Autodesk Inventor part; units mm, degrees
(part 4 of 5)
sketch "Эскиз44" plane through (1.5, 0, 0) normal (1, 0, 0) x (0, 0, -1)
  arc A0 (42, 27.152) -> (40, 25.152) centre (42, 25.152) ccw projected
  line L0 (40, 25.152) -> (40, 3) projected
  arc A1 (37, 0) -> (40, 3) centre (37, 3) ccw projected
  line L1 (37, 0) -> (-7, 0) projected
  arc A2 (-10, 3) -> (-7, 0) centre (-7, 3) ccw projected
  line L2 (-10, 3) -> (-10, 160) projected
  arc A3 (-7, 163) -> (-10, 160) centre (-7, 160) ccw projected
  line L3 (-7, 163) -> (37, 163) projected
  arc A4 (40, 160) -> (37, 163) centre (37, 160) ccw projected
  line L4 (40, 160) -> (40, 109.152) projected
  arc A5 (40, 109.152) -> (42, 107.152) centre (42, 109.152) ccw projected
  line L5 (42, 107.152) -> (54, 107.152) projected
  arc A6 (56, 105.152) -> (54, 107.152) centre (54, 105.152) ccw projected
  line L6 (56, 105.152) -> (56, 29.152) projected
  arc A7 (54, 27.152) -> (56, 29.152) centre (54, 29.152) ccw projected
  line L7 (54, 27.152) -> (42, 27.152) projected
  circle A8 centre (383.6, 368.9) radius 1.625 projected
  circle A9 centre (-13.6, 369) radius 1.625 projected
  circle A10 centre (383.6, 1.1) radius 1.625 projected
  circle A11 centre (-13.6, 1.1) radius 1.625 projected
  circle A12 centre (379.0468, 185.0848) radius 1.625 projected
  circle A13 centre (-9.0468, 185.0848) radius 1.625 projected
  circle A14 centre (379, 228) radius 1.625 projected
  circle A15 centre (-9, 228) radius 1.625 projected
  arc A16 (315.125, 369.3693) -> (315.125, 366.6307) centre (314.25, 368) ccw projected
  arc A17 (315.125, 366.6307) -> (315.125, 369.3693) centre (316, 368) ccw projected
  arc A18 (298.125, 229.3693) -> (298.125, 226.6307) centre (297.25, 228) ccw projected
  arc A19 (298.125, 226.6307) -> (298.125, 229.3693) centre (299, 228) ccw projected
  circle A20 centre (54, 228) radius 1.625 projected
  circle A21 centre (71, 142) radius 1.625 projected
  circle A22 centre (71, 2.0002) radius 1.625 projected
  circle A23 centre (54, 2.0002) radius 1.625 projected
  circle A24 centre (71, 368) radius 1.625 projected
  circle A25 centre (71, 228) radius 1.625 projected
  arc A26 (315.125, 143.3693) -> (315.125, 140.6307) centre (314.25, 142) ccw projected
  arc A27 (315.125, 140.6307) -> (315.125, 143.3693) centre (316, 142) ccw projected
  arc A28 (315.125, 229.3693) -> (315.125, 226.6307) centre (314.25, 228) ccw projected
  arc A29 (315.125, 226.6307) -> (315.125, 229.3693) centre (316, 228) ccw projected
  circle A30 centre (183.175, 129.0059) radius 1.85 projected
  arc A31 (298.125, 369.3693) -> (298.125, 366.6307) centre (297.25, 368) ccw projected
  arc A32 (298.125, 366.6307) -> (298.125, 369.3693) centre (299, 368) ccw projected
  arc A33 (315.125, 3.3695) -> (315.125, 0.6309) centre (314.25, 2.0002) ccw projected
  arc A34 (315.125, 0.6309) -> (315.125, 3.3695) centre (316, 2.0002) ccw projected
  circle A35 centre (54, 142) radius 1.625 projected
  circle A36 centre (54, 368) radius 1.625 projected
  arc A37 (298.125, 3.3695) -> (298.125, 0.6309) centre (297.25, 2.0002) ccw projected
  arc A38 (298.125, 0.6309) -> (298.125, 3.3695) centre (299, 2.0002) ccw projected
  arc A39 (298.125, 143.3693) -> (298.125, 140.6307) centre (297.25, 142) ccw projected
  arc A40 (298.125, 140.6307) -> (298.125, 143.3693) centre (299, 142) ccw projected
  arc A41 (185, 193.309) -> (185, 192.7028) centre (183.175, 193.0059) ccw projected
  line L8 (185, 193.309) -> (185, 192.7028) projected
  line L9 (14.5, 247.5001) -> (35, 247.5001) projected
  arc A42 (38, 244.5001) -> (35, 247.5001) centre (35, 244.5001) ccw projected
  line L10 (38, 244.5001) -> (38, 185.5001) projected
  arc A43 (35, 182.5001) -> (38, 185.5001) centre (35, 185.5001) ccw projected
  line L11 (35, 182.5001) -> (14.5, 182.5001) projected
  arc A44 (11.5, 185.5001) -> (14.5, 182.5001) centre (14.5, 185.5001) ccw projected
  line L12 (11.5, 185.5001) -> (11.5, 244.5001) projected
  arc A45 (14.5, 247.5001) -> (11.5, 244.5001) centre (14.5, 244.5001) ccw projected
  line L13 (358.5, 244.5001) -> (358.5, 185.5001) projected
  arc A46 (355.5, 182.5001) -> (358.5, 185.5001) centre (355.5, 185.5001) ccw projected
  line L14 (355.5, 182.5001) -> (335, 182.5001) projected
  arc A47 (332, 185.5001) -> (335, 182.5001) centre (335, 185.5001) ccw projected
  line L15 (332, 185.5001) -> (332, 244.5001) projected
  arc A48 (335, 247.5001) -> (332, 244.5001) centre (335, 244.5001) ccw projected
  line L16 (335, 247.5001) -> (355.5, 247.5001) projected
  arc A49 (358.5, 244.5001) -> (355.5, 247.5001) centre (355.5, 244.5001) ccw projected
  line L17 (98.825, 226.3849) -> (98.825, 137.3849) projected
  arc A50 (95.825, 134.3849) -> (98.825, 137.3849) centre (95.825, 137.3849) ccw projected
  line L18 (95.825, 134.3849) -> (87.825, 134.3849) projected
  arc A51 (84.825, 137.3849) -> (87.825, 134.3849) centre (87.825, 137.3849) ccw projected
  line L19 (84.825, 137.3849) -> (84.825, 226.3849) projected
  arc A52 (87.825, 229.3849) -> (84.825, 226.3849) centre (87.825, 226.3849) ccw projected
  line L20 (87.825, 229.3849) -> (95.825, 229.3849) projected
  arc A53 (98.825, 226.3849) -> (95.825, 229.3849) centre (95.825, 226.3849) ccw projected
  circle A54 centre (124.375, 129.0059) radius 2 projected
  circle A55 centre (124.375, 193.0059) radius 2 projected
  circle A56 centre (217.25, 312.9941) radius 2.1 projected
  circle A57 centre (152.75, 57.0059) radius 2.1 projected
  circle A58 centre (152.75, 118.0059) radius 2.1 projected
  circle A59 centre (152.75, 312.9941) radius 2.1 projected
  circle A60 centre (217.25, 251.9941) radius 2.1 projected
  circle A61 centre (217.25, 57.0059) radius 2.1 projected
  circle A62 centre (217.25, 118.0059) radius 2.1 projected
  circle A63 centre (152.75, 251.9941) radius 2.1 projected
  line L21 (165, 44) -> (165, 8) projected
  arc A64 (162, 5) -> (165, 8) centre (162, 8) ccw projected
  line L22 (162, 5) -> (96, 5) projected
  arc A65 (93, 8) -> (96, 5) centre (96, 8) ccw projected
  line L23 (93, 8) -> (93, 44) projected
  arc A66 (96, 47) -> (93, 44) centre (96, 44) ccw projected
  line L24 (96, 47) -> (162, 47) projected
  arc A67 (165, 44) -> (162, 47) centre (162, 44) ccw projected
  circle A68 centre (319.1128, 165.0002) radius 2.1 projected
  circle A69 centre (287, 56.343) radius 2.1 projected
  circle A70 centre (50.8872, 165.0002) radius 2.1 projected
  circle A71 centre (173.9908, 56.343) radius 2.1 projected
  circle A72 centre (135.25, 60) radius 2.1 projected
  circle A73 centre (103, 60) radius 2.1 projected
  line L25 (226.25, 270.0041) -> (226.25, 298.657) projected
  arc A74 (228.25, 300.657) -> (226.25, 298.657) centre (228.25, 298.657) ccw projected
  line L26 (228.25, 300.657) -> (268.3252, 300.657) projected
  arc A75 (269.4885, 297.03) -> (268.3252, 300.657) centre (268.3252, 298.657) ccw projected
  line L27 (269.4885, 297.03) -> (229.4132, 268.3772) projected
  arc A76 (226.25, 270.0041) -> (229.4132, 268.3772) centre (228.25, 270.0041) ccw projected
  arc A77 (235.9248, 170.343) -> (234.7615, 166.7161) centre (235.9248, 168.343) ccw projected
  line L28 (235.9248, 170.343) -> (276, 170.343) projected
  arc A78 (278, 168.343) -> (276, 170.343) centre (276, 168.343) ccw projected
  line L29 (278, 168.343) -> (278, 139.6902) projected
  arc A79 (274.8368, 138.0633) -> (278, 139.6902) centre (276, 139.6902) ccw projected
  line L30 (274.8368, 138.0633) -> (234.7615, 166.7161) projected
  arc A80 (94, 106.343) -> (92, 104.343) centre (94, 104.343) ccw projected
  line L31 (94, 106.343) -> (134.0752, 106.343) projected
  arc A81 (135.2385, 102.7161) -> (134.0752, 106.343) centre (134.0752, 104.343) ccw projected
  line L32 (135.2385, 102.7161) -> (95.1632, 74.0633) projected
  arc A82 (92, 75.6902) -> (95.1632, 74.0633) centre (94, 75.6902) ccw projected
  line L33 (92, 75.6902) -> (92, 104.343) projected
  arc A83 (92, 265.657) -> (94, 263.657) centre (94, 265.657) ccw projected
  line L34 (92, 265.657) -> (92, 294.3098) projected
  arc A84 (95.1632, 295.9367) -> (92, 294.3098) centre (94, 294.3098) ccw projected
  line L35 (95.1632, 295.9367) -> (135.2385, 267.2839) projected
  arc A85 (134.0752, 263.657) -> (135.2385, 267.2839) centre (134.0752, 265.657) ccw projected
  line L36 (134.0752, 263.657) -> (94, 263.657) projected
  arc A86 (130.725, 206.0059) -> (132.725, 204.0059) centre (132.725, 206.0059) ccw projected
  line L37 (130.725, 206.0059) -> (130.725, 234.2716) projected
  arc A87 (133.9769, 235.8314) -> (130.725, 234.2716) centre (132.725, 234.2716) ccw projected
  line L38 (133.9769, 235.8314) -> (169.1945, 207.5656) projected
  arc A88 (167.9426, 204.0059) -> (169.1945, 207.5656) centre (167.9426, 206.0059) ccw projected
  line L39 (167.9426, 204.0059) -> (132.725, 204.0059) projected
  arc A89 (226.25, 71.343) -> (228.25, 69.343) centre (228.25, 71.343) ccw projected
  line L40 (226.25, 71.343) -> (226.25, 99.9959) projected
  arc A90 (229.4132, 101.6228) -> (226.25, 99.9959) centre (228.25, 99.9959) ccw projected
  line L41 (229.4132, 101.6228) -> (269.4885, 72.97) projected
  arc A91 (268.3252, 69.343) -> (269.4885, 72.97) centre (268.3252, 71.343) ccw projected
  line L42 (268.3252, 69.343) -> (228.25, 69.343) projected
  arc A92 (226.25, 201.657) -> (228.25, 199.657) centre (228.25, 201.657) ccw projected
  line L43 (226.25, 201.657) -> (226.25, 230.3098) projected
  arc A93 (229.4132, 231.9367) -> (226.25, 230.3098) centre (228.25, 230.3098) ccw projected
  line L44 (229.4132, 231.9367) -> (269.4885, 203.2839) projected
  arc A94 (268.3252, 199.657) -> (269.4885, 203.2839) centre (268.3252, 201.657) ccw projected
  line L45 (268.3252, 199.657) -> (228.25, 199.657) projected
  arc A95 (278, 294.3098) -> (274.8368, 295.9367) centre (276, 294.3098) ccw projected
  line L46 (278, 294.3098) -> (278, 265.657) projected
  arc A96 (276, 263.657) -> (278, 265.657) centre (276, 265.657) ccw projected
  line L47 (276, 263.657) -> (235.9248, 263.657) projected
  arc A97 (234.7615, 267.2839) -> (235.9248, 263.657) centre (235.9248, 265.657) ccw projected
  line L48 (234.7615, 267.2839) -> (274.8368, 295.9367) projected
  arc A98 (226.25, 135.343) -> (228.25, 133.343) centre (228.25, 135.343) ccw projected
  line L49 (226.25, 135.343) -> (226.25, 163.9959) projected
  arc A99 (229.4132, 165.6228) -> (226.25, 163.9959) centre (228.25, 163.9959) ccw projected
  line L50 (229.4132, 165.6228) -> (269.4885, 136.97) projected
  arc A100 (268.3252, 133.343) -> (269.4885, 136.97) centre (268.3252, 135.343) ccw projected
  line L51 (268.3252, 133.343) -> (228.25, 133.343) projected
  arc A101 (143.75, 99.9959) -> (140.5868, 101.6228) centre (141.75, 99.9959) ccw projected
  line L52 (143.75, 99.9959) -> (143.75, 71.343) projected
  arc A102 (141.75, 69.343) -> (143.75, 71.343) centre (141.75, 71.343) ccw projected
  line L53 (141.75, 69.343) -> (101.6748, 69.343) projected
  arc A103 (100.5115, 72.97) -> (101.6748, 69.343) centre (101.6748, 71.343) ccw projected
  line L54 (100.5115, 72.97) -> (140.5868, 101.6228) projected
  arc A104 (143.75, 298.657) -> (141.75, 300.657) centre (141.75, 298.657) ccw projected
  line L55 (143.75, 298.657) -> (143.75, 270.0041) projected
  arc A105 (140.5868, 268.3772) -> (143.75, 270.0041) centre (141.75, 270.0041) ccw projected
  line L56 (140.5868, 268.3772) -> (100.5115, 297.03) projected
  arc A106 (101.6748, 300.657) -> (100.5115, 297.03) centre (101.6748, 298.657) ccw projected
  line L57 (101.6748, 300.657) -> (141.75, 300.657) projected
  line L58 (176.825, 239.0059) -> (176.825, 210.7401) projected
  arc A107 (173.5731, 209.1803) -> (176.825, 210.7401) centre (174.825, 210.7401) ccw projected
  line L59 (173.5731, 209.1803) -> (138.3555, 237.4461) projected
  arc A108 (139.6074, 241.0059) -> (138.3555, 237.4461) centre (139.6074, 239.0059) ccw projected
  line L60 (139.6074, 241.0059) -> (174.825, 241.0059) projected
  arc A109 (176.825, 239.0059) -> (174.825, 241.0059) centre (174.825, 239.0059) ccw projected
  line L61 (278, 104.343) -> (278, 75.6902) projected
  arc A110 (274.8368, 74.0633) -> (278, 75.6902) centre (276, 75.6902) ccw projected
  line L62 (274.8368, 74.0633) -> (234.7615, 102.7161) projected
  arc A111 (235.9248, 106.343) -> (234.7615, 102.7161) centre (235.9248, 104.343) ccw projected
  line L63 (235.9248, 106.343) -> (276, 106.343) projected
  arc A112 (278, 104.343) -> (276, 106.343) centre (276, 104.343) ccw projected
  arc A113 (278, 234.657) -> (276, 236.657) centre (276, 234.657) ccw projected
  line L64 (278, 234.657) -> (278, 206.0041) projected
  arc A114 (274.8368, 204.3772) -> (278, 206.0041) centre (276, 206.0041) ccw projected
  line L65 (274.8368, 204.3772) -> (234.7615, 233.03) projected
  arc A115 (235.9248, 236.657) -> (234.7615, 233.03) centre (235.9248, 234.657) ccw projected
  line L66 (235.9248, 236.657) -> (276, 236.657) projected
  arc A116 (295, 375) -> (292, 372) centre (295, 372) ccw projected
  line L67 (292, 372) -> (292, 323.5966) projected
  arc A117 (289, 320.5966) -> (292, 323.5966) centre (289, 323.5966) ccw projected
  line L68 (289, 320.5966) -> (81, 320.5966) projected
  arc A118 (78, 323.5966) -> (81, 320.5966) centre (81, 323.5966) ccw projected
  line L69 (78, 323.5966) -> (78, 372) projected
  arc A119 (78, 372) -> (75, 375) centre (75, 372) ccw projected
  line L70 (75, 375) -> (-15, 375) projected
  arc A120 (-15, 375) -> (-18, 372) centre (-15, 372) ccw projected
  line L71 (-18, 372) -> (-18, -2) projected
  arc A121 (-18, -2) -> (-15, -5) centre (-15, -2) ccw projected
  line L72 (-15, -5) -> (385, -5) projected
  arc A122 (385, -5) -> (388, -2) centre (385, -2) ccw projected
  line L73 (388, -2) -> (388, 372) projected
  arc A123 (388, 372) -> (385, 375) centre (385, 372) ccw projected
  line L74 (385, 375) -> (295, 375) projected
  arc A124 (40, 344.848) -> (42, 342.848) centre (42, 344.848) ccw projected
  line L75 (42, 342.848) -> (54, 342.848) projected
  arc A125 (56, 340.848) -> (54, 342.848) centre (54, 340.848) ccw projected
  line L76 (56, 340.848) -> (56, 264.848) projected
  arc A126 (54, 262.848) -> (56, 264.848) centre (54, 264.848) ccw projected
  line L77 (54, 262.848) -> (-8, 262.848) projected
  arc A127 (-10, 264.848) -> (-8, 262.848) centre (-8, 264.848) ccw projected
  line L78 (-10, 264.848) -> (-10, 367) projected
  arc A128 (-7, 370) -> (-10, 367) centre (-7, 367) ccw projected
  line L79 (-7, 370) -> (37, 370) projected
  arc A129 (40, 367) -> (37, 370) centre (37, 367) ccw projected
  line L80 (40, 367) -> (40, 344.848) projected
  line L81 (377, 0) -> (333, 0) projected
  arc A130 (330, 3) -> (333, 0) centre (333, 3) ccw projected
  line L82 (330, 3) -> (330, 28.152) projected
  arc A131 (330, 28.152) -> (327, 31.152) centre (327, 28.152) ccw projected
  line L83 (327, 31.152) -> (321, 31.152) projected
  arc A132 (318, 34.152) -> (321, 31.152) centre (321, 34.152) ccw projected
  line L84 (318, 34.152) -> (318, 100.152) projected
  arc A133 (321, 103.152) -> (318, 100.152) centre (321, 100.152) ccw projected
  line L85 (321, 103.152) -> (327, 103.152) projected
  arc A134 (327, 103.152) -> (330, 106.152) centre (327, 106.152) ccw projected
  line L86 (330, 106.152) -> (330, 160) projected
  arc A135 (333, 163) -> (330, 160) centre (333, 160) ccw projected
  line L87 (333, 163) -> (377, 163) projected
  arc A136 (380, 160) -> (377, 163) centre (377, 160) ccw projected
  line L88 (380, 160) -> (380, 3) projected
  arc A137 (377, 0) -> (380, 3) centre (377, 3) ccw projected
  line L89 (377, 266.848) -> (321, 266.848) projected
  arc A138 (318, 269.848) -> (321, 266.848) centre (321, 269.848) ccw projected
  line L90 (318, 269.848) -> (318, 335.848) projected
  arc A139 (321, 338.848) -> (318, 335.848) centre (321, 335.848) ccw projected
  line L91 (321, 338.848) -> (327, 338.848) projected
  arc A140 (327, 338.848) -> (330, 341.848) centre (327, 341.848) ccw projected
  line L92 (330, 341.848) -> (330, 367) projected
  arc A141 (333, 370) -> (330, 367) centre (333, 367) ccw projected
  line L93 (333, 370) -> (377, 370) projected
  arc A142 (380, 367) -> (377, 370) centre (377, 367) ccw projected
  line L94 (380, 367) -> (380, 269.848) projected
  arc A143 (377, 266.848) -> (380, 269.848) centre (377, 269.848) ccw projected
  circle A144 centre (314.25, 368) radius 1.625
  circle A145 centre (297.25, 368) radius 1.625
  circle A146 centre (297.25, 228) radius 1.625
  circle A147 centre (314.25, 228) radius 1.625
  circle A148 centre (297.25, 142) radius 1.625
  circle A149 centre (314.25, 142) radius 1.625
  circle A150 centre (297.25, 2.0002) radius 1.625
  circle A151 centre (314.25, 2.0002) radius 1.625
  point P0 (0, 0)
  point P1 (315.125, 0.6309)
  point P2 (315.125, 3.3695)
  point P3 (298.125, 0.6309)
  point P4 (298.125, 3.3695)
  point P5 (315.125, 226.6307)
  point P6 (315.125, 229.3693)
  point P7 (298.125, 226.6307)
  point P8 (298.125, 229.3693)
  constraints: 8 centre point, 1 coincident, 1 concentric
extrude "Выдавливание38" add sketch "Эскиз44" against normal up to surface (1.5 mm away) contours A17 A144 | A19 A146 | A27 A149 | A29 A147 | A32 A145 | A34 A151 | A38 A150 | A40 A148
ref_plane "РабПлоскость2" through (1.5, -2, -185) normal (0, 0, -1) x (-1, 0, 0)
mirror "Зеркальное отражение1" about plane through (1.5, -2, -185) normal (0, 0, -1) of "Выдавливание37"
sketch "Эскиз45" plane through (1.5, 0, 0) normal (1, 0, 0) x (0, 0, -1)
  arc A0 (42, 27.152) -> (40, 25.152) centre (42, 25.152) ccw projected
  line L0 (40, 25.152) -> (40, 3) projected
  arc A1 (37, 0) -> (40, 3) centre (37, 3) ccw projected
  line L1 (37, 0) -> (-7, 0) projected
  arc A2 (-10, 3) -> (-7, 0) centre (-7, 3) ccw projected
  line L2 (-10, 3) -> (-10, 160) projected
  arc A3 (-7, 163) -> (-10, 160) centre (-7, 160) ccw projected
  line L3 (-7, 163) -> (37, 163) projected
  arc A4 (40, 160) -> (37, 163) centre (37, 160) ccw projected
  line L4 (40, 160) -> (40, 109.152) projected
  arc A5 (40, 109.152) -> (42, 107.152) centre (42, 109.152) ccw projected
  line L5 (42, 107.152) -> (54, 107.152) projected
  arc A6 (56, 105.152) -> (54, 107.152) centre (54, 105.152) ccw projected
  line L6 (56, 105.152) -> (56, 29.152) projected
  arc A7 (54, 27.152) -> (56, 29.152) centre (54, 29.152) ccw projected
  line L7 (54, 27.152) -> (42, 27.152) projected
  circle A8 centre (383.6, 368.9) radius 1.625 projected
  circle A9 centre (-13.6, 369) radius 1.625 projected
  circle A10 centre (383.6, 1.1) radius 1.625 projected
  circle A11 centre (-13.6, 1.1) radius 1.625 projected
  circle A12 centre (379.0468, 185.0848) radius 1.625 projected
  circle A13 centre (-9.0468, 185.0848) radius 1.625 projected
  circle A14 centre (379, 228) radius 1.625 projected
  circle A15 centre (-9, 228) radius 1.625 projected
  circle A16 centre (314.25, 368) radius 1.625 projected
  circle A17 centre (297.25, 228) radius 1.625 projected
  arc A18 (54.875, 226.6307) -> (54.875, 229.3693) centre (55.75, 228) ccw projected
  arc A19 (54.875, 229.3693) -> (54.875, 226.6307) centre (54, 228) ccw projected
  arc A20 (71.875, 140.6307) -> (71.875, 143.3693) centre (72.75, 142) ccw projected
  arc A21 (71.875, 143.3693) -> (71.875, 140.6307) centre (71, 142) ccw projected
  arc A22 (71.875, 0.6309) -> (71.875, 3.3695) centre (72.75, 2.0002) ccw projected
  arc A23 (71.875, 3.3695) -> (71.875, 0.6309) centre (71, 2.0002) ccw projected
  arc A24 (54.875, 0.6309) -> (54.875, 3.3695) centre (55.75, 2.0002) ccw projected
  arc A25 (54.875, 3.3695) -> (54.875, 0.6309) centre (54, 2.0002) ccw projected
  arc A26 (71.875, 366.6307) -> (71.875, 369.3693) centre (72.75, 368) ccw projected
  arc A27 (71.875, 369.3693) -> (71.875, 366.6307) centre (71, 368) ccw projected
  arc A28 (71.875, 226.6307) -> (71.875, 229.3693) centre (72.75, 228) ccw projected
  arc A29 (71.875, 229.3693) -> (71.875, 226.6307) centre (71, 228) ccw projected
  circle A30 centre (314.25, 142) radius 1.625 projected
  circle A31 centre (314.25, 228) radius 1.625 projected
  circle A32 centre (183.175, 129.0059) radius 1.85 projected
  circle A33 centre (297.25, 368) radius 1.625 projected
  circle A34 centre (314.25, 2.0002) radius 1.625 projected
  arc A35 (54.875, 140.6307) -> (54.875, 143.3693) centre (55.75, 142) ccw projected
  arc A36 (54.875, 143.3693) -> (54.875, 140.6307) centre (54, 142) ccw projected
  arc A37 (54.875, 366.6307) -> (54.875, 369.3693) centre (55.75, 368) ccw projected
  arc A38 (54.875, 369.3693) -> (54.875, 366.6307) centre (54, 368) ccw projected
  circle A39 centre (297.25, 2.0002) radius 1.625 projected
  circle A40 centre (297.25, 142) radius 1.625 projected
  arc A41 (185, 193.309) -> (185, 192.7028) centre (183.175, 193.0059) ccw projected
  line L8 (185, 193.309) -> (185, 192.7028) projected
  line L9 (14.5, 247.5001) -> (35, 247.5001) projected
  arc A42 (38, 244.5001) -> (35, 247.5001) centre (35, 244.5001) ccw projected
  line L10 (38, 244.5001) -> (38, 185.5001) projected
  arc A43 (35, 182.5001) -> (38, 185.5001) centre (35, 185.5001) ccw projected
  line L11 (35, 182.5001) -> (14.5, 182.5001) projected
  arc A44 (11.5, 185.5001) -> (14.5, 182.5001) centre (14.5, 185.5001) ccw projected
  line L12 (11.5, 185.5001) -> (11.5, 244.5001) projected
  arc A45 (14.5, 247.5001) -> (11.5, 244.5001) centre (14.5, 244.5001) ccw projected
  line L13 (358.5, 244.5001) -> (358.5, 185.5001) projected
  arc A46 (355.5, 182.5001) -> (358.5, 185.5001) centre (355.5, 185.5001) ccw projected
  line L14 (355.5, 182.5001) -> (335, 182.5001) projected
  arc A47 (332, 185.5001) -> (335, 182.5001) centre (335, 185.5001) ccw projected
  line L15 (332, 185.5001) -> (332, 244.5001) projected
  arc A48 (335, 247.5001) -> (332, 244.5001) centre (335, 244.5001) ccw projected
  line L16 (335, 247.5001) -> (355.5, 247.5001) projected
  arc A49 (358.5, 244.5001) -> (355.5, 247.5001) centre (355.5, 244.5001) ccw projected
  line L17 (98.825, 226.3849) -> (98.825, 137.3849) projected
  arc A50 (95.825, 134.3849) -> (98.825, 137.3849) centre (95.825, 137.3849) ccw projected
  line L18 (95.825, 134.3849) -> (87.825, 134.3849) projected
  arc A51 (84.825, 137.3849) -> (87.825, 134.3849) centre (87.825, 137.3849) ccw projected
  line L19 (84.825, 137.3849) -> (84.825, 226.3849) projected
  arc A52 (87.825, 229.3849) -> (84.825, 226.3849) centre (87.825, 226.3849) ccw projected
  line L20 (87.825, 229.3849) -> (95.825, 229.3849) projected
  arc A53 (98.825, 226.3849) -> (95.825, 229.3849) centre (95.825, 226.3849) ccw projected
  circle A54 centre (124.375, 129.0059) radius 2 projected
  circle A55 centre (124.375, 193.0059) radius 2 projected
  circle A56 centre (217.25, 312.9941) radius 2.1 projected
  circle A57 centre (152.75, 57.0059) radius 2.1 projected
  circle A58 centre (152.75, 118.0059) radius 2.1 projected
  circle A59 centre (152.75, 312.9941) radius 2.1 projected
  circle A60 centre (217.25, 251.9941) radius 2.1 projected
  circle A61 centre (217.25, 57.0059) radius 2.1 projected
  circle A62 centre (217.25, 118.0059) radius 2.1 projected
  circle A63 centre (152.75, 251.9941) radius 2.1 projected
  line L21 (165, 44) -> (165, 8) projected
  arc A64 (162, 5) -> (165, 8) centre (162, 8) ccw projected
  line L22 (162, 5) -> (96, 5) projected
  arc A65 (93, 8) -> (96, 5) centre (96, 8) ccw projected
  line L23 (93, 8) -> (93, 44) projected
  arc A66 (96, 47) -> (93, 44) centre (96, 44) ccw projected
  line L24 (96, 47) -> (162, 47) projected
  arc A67 (165, 44) -> (162, 47) centre (162, 44) ccw projected
  circle A68 centre (319.1128, 165.0002) radius 2.1 projected
  circle A69 centre (287, 56.343) radius 2.1 projected
  circle A70 centre (50.8872, 165.0002) radius 2.1 projected
  circle A71 centre (173.9908, 56.343) radius 2.1 projected
  circle A72 centre (135.25, 60) radius 2.1 projected
  circle A73 centre (103, 60) radius 2.1 projected
  line L25 (226.25, 270.0041) -> (226.25, 298.657) projected
  arc A74 (228.25, 300.657) -> (226.25, 298.657) centre (228.25, 298.657) ccw projected
  line L26 (228.25, 300.657) -> (268.3252, 300.657) projected
  arc A75 (269.4885, 297.03) -> (268.3252, 300.657) centre (268.3252, 298.657) ccw projected
  line L27 (269.4885, 297.03) -> (229.4132, 268.3772) projected
  arc A76 (226.25, 270.0041) -> (229.4132, 268.3772) centre (228.25, 270.0041) ccw projected
  arc A77 (235.9248, 170.343) -> (234.7615, 166.7161) centre (235.9248, 168.343) ccw projected
  line L28 (235.9248, 170.343) -> (276, 170.343) projected
  arc A78 (278, 168.343) -> (276, 170.343) centre (276, 168.343) ccw projected
  line L29 (278, 168.343) -> (278, 139.6902) projected
  arc A79 (274.8368, 138.0633) -> (278, 139.6902) centre (276, 139.6902) ccw projected
  line L30 (274.8368, 138.0633) -> (234.7615, 166.7161) projected
  arc A80 (94, 106.343) -> (92, 104.343) centre (94, 104.343) ccw projected
  line L31 (94, 106.343) -> (134.0752, 106.343) projected
  arc A81 (135.2385, 102.7161) -> (134.0752, 106.343) centre (134.0752, 104.343) ccw projected
  line L32 (135.2385, 102.7161) -> (95.1632, 74.0633) projected
  arc A82 (92, 75.6902) -> (95.1632, 74.0633) centre (94, 75.6902) ccw projected
  line L33 (92, 75.6902) -> (92, 104.343) projected
  arc A83 (92, 265.657) -> (94, 263.657) centre (94, 265.657) ccw projected
  line L34 (92, 265.657) -> (92, 294.3098) projected
  arc A84 (95.1632, 295.9367) -> (92, 294.3098) centre (94, 294.3098) ccw projected
  line L35 (95.1632, 295.9367) -> (135.2385, 267.2839) projected
  arc A85 (134.0752, 263.657) -> (135.2385, 267.2839) centre (134.0752, 265.657) ccw projected
  line L36 (134.0752, 263.657) -> (94, 263.657) projected
  arc A86 (130.725, 206.0059) -> (132.725, 204.0059) centre (132.725, 206.0059) ccw projected
  line L37 (130.725, 206.0059) -> (130.725, 234.2716) projected
  arc A87 (133.9769, 235.8314) -> (130.725, 234.2716) centre (132.725, 234.2716) ccw projected
  line L38 (133.9769, 235.8314) -> (169.1945, 207.5656) projected
  arc A88 (167.9426, 204.0059) -> (169.1945, 207.5656) centre (167.9426, 206.0059) ccw projected
  line L39 (167.9426, 204.0059) -> (132.725, 204.0059) projected
  arc A89 (226.25, 71.343) -> (228.25, 69.343) centre (228.25, 71.343) ccw projected
  line L40 (226.25, 71.343) -> (226.25, 99.9959) projected
  arc A90 (229.4132, 101.6228) -> (226.25, 99.9959) centre (228.25, 99.9959) ccw projected
  line L41 (229.4132, 101.6228) -> (269.4885, 72.97) projected
  arc A91 (268.3252, 69.343) -> (269.4885, 72.97) centre (268.3252, 71.343) ccw projected
  line L42 (268.3252, 69.343) -> (228.25, 69.343) projected
  arc A92 (226.25, 201.657) -> (228.25, 199.657) centre (228.25, 201.657) ccw projected
  line L43 (226.25, 201.657) -> (226.25, 230.3098) projected
  arc A93 (229.4132, 231.9367) -> (226.25, 230.3098) centre (228.25, 230.3098) ccw projected
  line L44 (229.4132, 231.9367) -> (269.4885, 203.2839) projected
  arc A94 (268.3252, 199.657) -> (269.4885, 203.2839) centre (268.3252, 201.657) ccw projected
  line L45 (268.3252, 199.657) -> (228.25, 199.657) projected
  arc A95 (278, 294.3098) -> (274.8368, 295.9367) centre (276, 294.3098) ccw projected
  line L46 (278, 294.3098) -> (278, 265.657) projected
  arc A96 (276, 263.657) -> (278, 265.657) centre (276, 265.657) ccw projected
  line L47 (276, 263.657) -> (235.9248, 263.657) projected
  arc A97 (234.7615, 267.2839) -> (235.9248, 263.657) centre (235.9248, 265.657) ccw projected
  line L48 (234.7615, 267.2839) -> (274.8368, 295.9367) projected
  arc A98 (226.25, 135.343) -> (228.25, 133.343) centre (228.25, 135.343) ccw projected
  line L49 (226.25, 135.343) -> (226.25, 163.9959) projected
  arc A99 (229.4132, 165.6228) -> (226.25, 163.9959) centre (228.25, 163.9959) ccw projected
  line L50 (229.4132, 165.6228) -> (269.4885, 136.97) projected
  arc A100 (268.3252, 133.343) -> (269.4885, 136.97) centre (268.3252, 135.343) ccw projected
  line L51 (268.3252, 133.343) -> (228.25, 133.343) projected
  arc A101 (143.75, 99.9959) -> (140.5868, 101.6228) centre (141.75, 99.9959) ccw projected
  line L52 (143.75, 99.9959) -> (143.75, 71.343) projected
  arc A102 (141.75, 69.343) -> (143.75, 71.343) centre (141.75, 71.343) ccw projected
  line L53 (141.75, 69.343) -> (101.6748, 69.343) projected
  arc A103 (100.5115, 72.97) -> (101.6748, 69.343) centre (101.6748, 71.343) ccw projected
  line L54 (100.5115, 72.97) -> (140.5868, 101.6228) projected
  arc A104 (143.75, 298.657) -> (141.75, 300.657) centre (141.75, 298.657) ccw projected
  line L55 (143.75, 298.657) -> (143.75, 270.0041) projected
  arc A105 (140.5868, 268.3772) -> (143.75, 270.0041) centre (141.75, 270.0041) ccw projected
  line L56 (140.5868, 268.3772) -> (100.5115, 297.03) projected
  arc A106 (101.6748, 300.657) -> (100.5115, 297.03) centre (101.6748, 298.657) ccw projected
  line L57 (101.6748, 300.657) -> (141.75, 300.657) projected
  line L58 (176.825, 239.0059) -> (176.825, 210.7401) projected
  arc A107 (173.5731, 209.1803) -> (176.825, 210.7401) centre (174.825, 210.7401) ccw projected
  line L59 (173.5731, 209.1803) -> (138.3555, 237.4461) projected
  arc A108 (139.6074, 241.0059) -> (138.3555, 237.4461) centre (139.6074, 239.0059) ccw projected
  line L60 (139.6074, 241.0059) -> (174.825, 241.0059) projected
  arc A109 (176.825, 239.0059) -> (174.825, 241.0059) centre (174.825, 239.0059) ccw projected
  line L61 (278, 104.343) -> (278, 75.6902) projected
  arc A110 (274.8368, 74.0633) -> (278, 75.6902) centre (276, 75.6902) ccw projected
  line L62 (274.8368, 74.0633) -> (234.7615, 102.7161) projected
  arc A111 (235.9248, 106.343) -> (234.7615, 102.7161) centre (235.9248, 104.343) ccw projected
  line L63 (235.9248, 106.343) -> (276, 106.343) projected
  arc A112 (278, 104.343) -> (276, 106.343) centre (276, 104.343) ccw projected
  arc A113 (278, 234.657) -> (276, 236.657) centre (276, 234.657) ccw projected
  line L64 (278, 234.657) -> (278, 206.0041) projected
  arc A114 (274.8368, 204.3772) -> (278, 206.0041) centre (276, 206.0041) ccw projected
  line L65 (274.8368, 204.3772) -> (234.7615, 233.03) projected
  arc A115 (235.9248, 236.657) -> (234.7615, 233.03) centre (235.9248, 234.657) ccw projected
  line L66 (235.9248, 236.657) -> (276, 236.657) projected
  arc A116 (295, 375) -> (292, 372) centre (295, 372) ccw projected
  line L67 (292, 372) -> (292, 323.5966) projected
  arc A117 (289, 320.5966) -> (292, 323.5966) centre (289, 323.5966) ccw projected
  line L68 (289, 320.5966) -> (81, 320.5966) projected
  arc A118 (78, 323.5966) -> (81, 320.5966) centre (81, 323.5966) ccw projected
  line L69 (78, 323.5966) -> (78, 372) projected
  arc A119 (78, 372) -> (75, 375) centre (75, 372) ccw projected
  line L70 (75, 375) -> (-15, 375) projected
  arc A120 (-15, 375) -> (-18, 372) centre (-15, 372) ccw projected
  line L71 (-18, 372) -> (-18, -2) projected
  arc A121 (-18, -2) -> (-15, -5) centre (-15, -2) ccw projected
  line L72 (-15, -5) -> (385, -5) projected
  arc A122 (385, -5) -> (388, -2) centre (385, -2) ccw projected
  line L73 (388, -2) -> (388, 372) projected
  arc A123 (388, 372) -> (385, 375) centre (385, 372) ccw projected
  line L74 (385, 375) -> (295, 375) projected
  arc A124 (40, 344.848) -> (42, 342.848) centre (42, 344.848) ccw projected
  line L75 (42, 342.848) -> (54, 342.848) projected
  arc A125 (56, 340.848) -> (54, 342.848) centre (54, 340.848) ccw projected
  line L76 (56, 340.848) -> (56, 264.848) projected
  arc A126 (54, 262.848) -> (56, 264.848) centre (54, 264.848) ccw projected
  line L77 (54, 262.848) -> (-8, 262.848) projected
  arc A127 (-10, 264.848) -> (-8, 262.848) centre (-8, 264.848) ccw projected
  line L78 (-10, 264.848) -> (-10, 367) projected
  arc A128 (-7, 370) -> (-10, 367) centre (-7, 367) ccw projected
  line L79 (-7, 370) -> (37, 370) projected
  arc A129 (40, 367) -> (37, 370) centre (37, 367) ccw projected
  line L80 (40, 367) -> (40, 344.848) projected
  line L81 (377, 0) -> (333, 0) projected
  arc A130 (330, 3) -> (333, 0) centre (333, 3) ccw projected
  line L82 (330, 3) -> (330, 28.152) projected
  arc A131 (330, 28.152) -> (327, 31.152) centre (327, 28.152) ccw projected
  line L83 (327, 31.152) -> (321, 31.152) projected
  arc A132 (318, 34.152) -> (321, 31.152) centre (321, 34.152) ccw projected
  line L84 (318, 34.152) -> (318, 100.152) projected
  arc A133 (321, 103.152) -> (318, 100.152) centre (321, 100.152) ccw projected
  line L85 (321, 103.152) -> (327, 103.152) projected
  arc A134 (327, 103.152) -> (330, 106.152) centre (327, 106.152) ccw projected
  line L86 (330, 106.152) -> (330, 160) projected
  arc A135 (333, 163) -> (330, 160) centre (333, 160) ccw projected
  line L87 (333, 163) -> (377, 163) projected
  arc A136 (380, 160) -> (377, 163) centre (377, 160) ccw projected
  line L88 (380, 160) -> (380, 3) projected
  arc A137 (377, 0) -> (380, 3) centre (377, 3) ccw projected
  line L89 (377, 266.848) -> (321, 266.848) projected
  arc A138 (318, 269.848) -> (321, 266.848) centre (321, 269.848) ccw projected
  line L90 (318, 269.848) -> (318, 335.848) projected
  arc A139 (321, 338.848) -> (318, 335.848) centre (321, 335.848) ccw projected
  line L91 (321, 338.848) -> (327, 338.848) projected
  arc A140 (327, 338.848) -> (330, 341.848) centre (327, 341.848) ccw projected
  line L92 (330, 341.848) -> (330, 367) projected
  arc A141 (333, 370) -> (330, 367) centre (333, 367) ccw projected
  line L93 (333, 370) -> (377, 370) projected
  arc A142 (380, 367) -> (377, 370) centre (377, 367) ccw projected
  line L94 (380, 367) -> (380, 269.848) projected
  arc A143 (377, 266.848) -> (380, 269.848) centre (377, 269.848) ccw projected
  circle A144 centre (72.75, 368) radius 1.625
  circle A145 centre (55.75, 368) radius 1.625
  circle A146 centre (72.75, 228) radius 1.625
  circle A147 centre (55.75, 228) radius 1.625
  circle A148 centre (72.75, 142) radius 1.625
  circle A149 centre (55.75, 142) radius 1.625
  circle A150 centre (72.75, 2.0002) radius 1.625
  circle A151 centre (55.75, 2.0002) radius 1.625
  line L95 (291, 320.5966) -> (291, 375)
  line L96 (291, 375) -> (79, 375)
  line L97 (81, 377) -> (81, 320.5966)
  line L98 (289, 320.5966) -> (81, 320.5966) projected
  line L99 (79, 320.5966) -> (79, 377)
  line L100 (79, 377) -> (293, 377)
  line L101 (293, 377) -> (293, 320.5966)
  point P0 (0, 0)
  point P1 (71.875, 0.6309)
  point P2 (71.875, 3.3695)
  point P3 (54.875, 0.6309)
  point P4 (54.875, 226.6307)
  point P5 (54.875, 229.3693)
  point P6 (71.875, 226.6307)
  point P7 (71.875, 229.3693)
  point P8 (54.875, 366.6307)
  point P9 (54.875, 369.3693)
  point P10 (81, 375)
  point P11 (78, 347.7983)
  point P12 (291, 321.3605)
  point P13 (79, 321.3605)
  dimension "d244" = 1
  dimension "d247" = 0
  dimension "d248" = 0
  dimension "d250" = 2
  constraints: 12 end point, 7 centre point, 4 point on line, 1 coincident, 1 midpoint, 1 parallel, 3 other
  measures "d244" distance between parallel lines of L67 L95
  measures "d247" distance between parallel lines of L70 L96
  measures "d248" angle of L69 L97
  measures "d250" distance between parallel lines of L97 L99
extrude "Выдавливание39" add sketch "Эскиз45" against normal up to surface (1.5 mm away) contours A19 A147 | A21 A148 | A23 A150 | A25 A151 | A27 A144 | A29 A146 | A36 A149 | A38 A145 | L25 A74 L26 A75 L27 A76 | L28 A78 L29 A79 L30 A77 | L31 A81 L32 A82 L33 A80 | L34 A84 L35 A85 L36 A83 | L37 A87 L38 A88 L39 A86 | L40 A90 L41 A91 L42 A89 | L43 A93 L44 A94 L45 A92 | L46 A96 L47 A97 L48 A95 | L49 A99 L50 A100 L51 A98 | L52 A102 L53 A103 L54 A101 | L55 A105 L56 A106 L57 A104 | L58 A107 L59 A108 L60 A109 | L61 A110 L62 A111 L63 A112 | L64 A114 L65 A115 L66 A113 | A117 L68 L97 L96 L95 | L97 A118 L99 L96
sketch "Эскиз46" plane through (1.5, 0, 0) normal (1, 0, 0) x (0, 0, -1)
  line L0 (289, 320.5966) -> (81, 320.5966) projected
  line L1 (79, 320.5966) -> (291, 320.5966)
  line L2 (291, 320.5966) -> (291, 375)
  line L3 (291, 375) -> (79, 375)
  line L4 (79, 375) -> (79, 320.5966)
  arc A0 (42, 27.152) -> (40, 25.152) centre (42, 25.152) ccw projected
  line L5 (40, 25.152) -> (40, 3) projected
  arc A1 (37, 0) -> (40, 3) centre (37, 3) ccw projected
  line L6 (37, 0) -> (-7, 0) projected
  arc A2 (-10, 3) -> (-7, 0) centre (-7, 3) ccw projected
  line L7 (-10, 3) -> (-10, 160) projected
  arc A3 (-7, 163) -> (-10, 160) centre (-7, 160) ccw projected
  line L8 (-7, 163) -> (37, 163) projected
  arc A4 (40, 160) -> (37, 163) centre (37, 160) ccw projected
  line L9 (40, 160) -> (40, 109.152) projected
  arc A5 (40, 109.152) -> (42, 107.152) centre (42, 109.152) ccw projected
  line L10 (42, 107.152) -> (54, 107.152) projected
  arc A6 (56, 105.152) -> (54, 107.152) centre (54, 105.152) ccw projected
  line L11 (56, 105.152) -> (56, 29.152) projected
  arc A7 (54, 27.152) -> (56, 29.152) centre (54, 29.152) ccw projected
  line L12 (54, 27.152) -> (42, 27.152) projected
  circle A8 centre (383.6, 368.9) radius 1.625 projected
  circle A9 centre (-13.6, 369) radius 1.625 projected
  circle A10 centre (383.6, 1.1) radius 1.625 projected
  circle A11 centre (-13.6, 1.1) radius 1.625 projected
  circle A12 centre (379.0468, 185.0848) radius 1.625 projected
  circle A13 centre (-9.0468, 185.0848) radius 1.625 projected
  circle A14 centre (379, 228) radius 1.625 projected
  circle A15 centre (-9, 228) radius 1.625 projected
  circle A16 centre (314.25, 368) radius 1.625 projected
  circle A17 centre (297.25, 228) radius 1.625 projected
  circle A18 centre (55.75, 228) radius 1.625 projected
  circle A19 centre (72.75, 142) radius 1.625 projected
  circle A20 centre (72.75, 2.0002) radius 1.625 projected
  circle A21 centre (55.75, 2.0002) radius 1.625 projected
  circle A22 centre (72.75, 368) radius 1.625 projected
  circle A23 centre (72.75, 228) radius 1.625 projected
  circle A24 centre (314.25, 142) radius 1.625 projected
  circle A25 centre (314.25, 228) radius 1.625 projected
  circle A26 centre (183.175, 129.0059) radius 1.85 projected
  circle A27 centre (297.25, 368) radius 1.625 projected
  circle A28 centre (314.25, 2.0002) radius 1.625 projected
  circle A29 centre (55.75, 142) radius 1.625 projected
  circle A30 centre (55.75, 368) radius 1.625 projected
  circle A31 centre (297.25, 2.0002) radius 1.625 projected
  circle A32 centre (297.25, 142) radius 1.625 projected
  arc A33 (185, 193.309) -> (185, 192.7028) centre (183.175, 193.0059) ccw projected
  line L13 (185, 193.309) -> (185, 192.7028) projected
  line L14 (14.5, 247.5001) -> (35, 247.5001) projected
  arc A34 (38, 244.5001) -> (35, 247.5001) centre (35, 244.5001) ccw projected
  line L15 (38, 244.5001) -> (38, 185.5001) projected
  arc A35 (35, 182.5001) -> (38, 185.5001) centre (35, 185.5001) ccw projected
  line L16 (35, 182.5001) -> (14.5, 182.5001) projected
  arc A36 (11.5, 185.5001) -> (14.5, 182.5001) centre (14.5, 185.5001) ccw projected
  line L17 (11.5, 185.5001) -> (11.5, 244.5001) projected
  arc A37 (14.5, 247.5001) -> (11.5, 244.5001) centre (14.5, 244.5001) ccw projected
  line L18 (358.5, 244.5001) -> (358.5, 185.5001) projected
  arc A38 (355.5, 182.5001) -> (358.5, 185.5001) centre (355.5, 185.5001) ccw projected
  line L19 (355.5, 182.5001) -> (335, 182.5001) projected
  arc A39 (332, 185.5001) -> (335, 182.5001) centre (335, 185.5001) ccw projected
  line L20 (332, 185.5001) -> (332, 244.5001) projected
  arc A40 (335, 247.5001) -> (332, 244.5001) centre (335, 244.5001) ccw projected
  line L21 (335, 247.5001) -> (355.5, 247.5001) projected
  arc A41 (358.5, 244.5001) -> (355.5, 247.5001) centre (355.5, 244.5001) ccw projected
  line L22 (98.825, 226.3849) -> (98.825, 137.3849) projected
  arc A42 (95.825, 134.3849) -> (98.825, 137.3849) centre (95.825, 137.3849) ccw projected
  line L23 (95.825, 134.3849) -> (87.825, 134.3849) projected
  arc A43 (84.825, 137.3849) -> (87.825, 134.3849) centre (87.825, 137.3849) ccw projected
  line L24 (84.825, 137.3849) -> (84.825, 226.3849) projected
  arc A44 (87.825, 229.3849) -> (84.825, 226.3849) centre (87.825, 226.3849) ccw projected
  line L25 (87.825, 229.3849) -> (95.825, 229.3849) projected
  arc A45 (98.825, 226.3849) -> (95.825, 229.3849) centre (95.825, 226.3849) ccw projected
  circle A46 centre (124.375, 129.0059) radius 2 projected
  circle A47 centre (124.375, 193.0059) radius 2 projected
  circle A48 centre (217.25, 312.9941) radius 2.1 projected
  circle A49 centre (152.75, 57.0059) radius 2.1 projected
  circle A50 centre (152.75, 118.0059) radius 2.1 projected
  circle A51 centre (152.75, 312.9941) radius 2.1 projected
  circle A52 centre (217.25, 251.9941) radius 2.1 projected
  circle A53 centre (217.25, 57.0059) radius 2.1 projected
  circle A54 centre (217.25, 118.0059) radius 2.1 projected
  circle A55 centre (152.75, 251.9941) radius 2.1 projected
  line L26 (165, 44) -> (165, 8) projected
  arc A56 (162, 5) -> (165, 8) centre (162, 8) ccw projected
  line L27 (162, 5) -> (96, 5) projected
  arc A57 (93, 8) -> (96, 5) centre (96, 8) ccw projected
  line L28 (93, 8) -> (93, 44) projected
  arc A58 (96, 47) -> (93, 44) centre (96, 44) ccw projected
  line L29 (96, 47) -> (162, 47) projected
  arc A59 (165, 44) -> (162, 47) centre (162, 44) ccw projected
  circle A60 centre (319.1128, 165.0002) radius 2.1 projected
  circle A61 centre (287, 56.343) radius 2.1 projected
  circle A62 centre (50.8872, 165.0002) radius 2.1 projected
  circle A63 centre (173.9908, 56.343) radius 2.1 projected
  circle A64 centre (135.25, 60) radius 2.1 projected
  circle A65 centre (103, 60) radius 2.1 projected
  arc A66 (295, 375) -> (292, 372) centre (295, 372) ccw projected
  line L30 (292, 372) -> (292, 323.5966) projected
  arc A67 (291, 321.3605) -> (292, 323.5966) centre (289, 323.5966) ccw projected
  arc A68 (78, 323.5966) -> (79, 321.3605) centre (81, 323.5966) ccw projected
  line L31 (78, 323.5966) -> (78, 372) projected
  arc A69 (78, 372) -> (75, 375) centre (75, 372) ccw projected
  line L32 (75, 375) -> (-15, 375) projected
  arc A70 (-15, 375) -> (-18, 372) centre (-15, 372) ccw projected
  line L33 (-18, 372) -> (-18, -2) projected
  arc A71 (-18, -2) -> (-15, -5) centre (-15, -2) ccw projected
  line L34 (-15, -5) -> (385, -5) projected
  arc A72 (385, -5) -> (388, -2) centre (385, -2) ccw projected
  line L35 (388, -2) -> (388, 372) projected
  arc A73 (388, 372) -> (385, 375) centre (385, 372) ccw projected
  line L36 (385, 375) -> (295, 375) projected
  arc A74 (40, 344.848) -> (42, 342.848) centre (42, 344.848) ccw projected
  line L37 (42, 342.848) -> (54, 342.848) projected
  arc A75 (56, 340.848) -> (54, 342.848) centre (54, 340.848) ccw projected
  line L38 (56, 340.848) -> (56, 264.848) projected
  arc A76 (54, 262.848) -> (56, 264.848) centre (54, 264.848) ccw projected
  line L39 (54, 262.848) -> (-8, 262.848) projected
  arc A77 (-10, 264.848) -> (-8, 262.848) centre (-8, 264.848) ccw projected
  line L40 (-10, 264.848) -> (-10, 367) projected
  arc A78 (-7, 370) -> (-10, 367) centre (-7, 367) ccw projected
  line L41 (-7, 370) -> (37, 370) projected
  arc A79 (40, 367) -> (37, 370) centre (37, 367) ccw projected
  line L42 (40, 367) -> (40, 344.848) projected
  line L43 (377, 0) -> (333, 0) projected
  arc A80 (330, 3) -> (333, 0) centre (333, 3) ccw projected
  line L44 (330, 3) -> (330, 28.152) projected
  arc A81 (330, 28.152) -> (327, 31.152) centre (327, 28.152) ccw projected
  line L45 (327, 31.152) -> (321, 31.152) projected
  arc A82 (318, 34.152) -> (321, 31.152) centre (321, 34.152) ccw projected
  line L46 (318, 34.152) -> (318, 100.152) projected
  arc A83 (321, 103.152) -> (318, 100.152) centre (321, 100.152) ccw projected
  line L47 (321, 103.152) -> (327, 103.152) projected
  arc A84 (327, 103.152) -> (330, 106.152) centre (327, 106.152) ccw projected
  line L48 (330, 106.152) -> (330, 160) projected
  arc A85 (333, 163) -> (330, 160) centre (333, 160) ccw projected
  line L49 (333, 163) -> (377, 163) projected
  arc A86 (380, 160) -> (377, 163) centre (377, 160) ccw projected
  line L50 (380, 160) -> (380, 3) projected
  arc A87 (377, 0) -> (380, 3) centre (377, 3) ccw projected
  line L51 (377, 266.848) -> (321, 266.848) projected
  arc A88 (318, 269.848) -> (321, 266.848) centre (321, 269.848) ccw projected
  line L52 (318, 269.848) -> (318, 335.848) projected
  arc A89 (321, 338.848) -> (318, 335.848) centre (321, 335.848) ccw projected
  line L53 (321, 338.848) -> (327, 338.848) projected
  arc A90 (327, 338.848) -> (330, 341.848) centre (327, 341.848) ccw projected
  line L54 (330, 341.848) -> (330, 367) projected
  arc A91 (333, 370) -> (330, 367) centre (333, 367) ccw projected
  line L55 (333, 370) -> (377, 370) projected
  arc A92 (380, 367) -> (377, 370) centre (377, 367) ccw projected
  line L56 (380, 367) -> (380, 269.848) projected
  arc A93 (377, 266.848) -> (380, 269.848) centre (377, 269.848) ccw projected
  line L57 (72.75, 142) -> (78.75, 142)
  line L58 (87.825, 134.3849) -> (78.75, 134.3849)
  line L59 (78.75, 134.3849) -> (78.75, 229.3849)
  line L60 (78.75, 229.3849) -> (87.825, 229.3849)
  line L61 (87.825, 229.3849) -> (87.825, 134.3849)
  line L62 (95.825, 134.3849) -> (100.825, 134.3849)
  line L63 (100.825, 134.3849) -> (100.825, 229.3849)
  line L64 (100.825, 229.3849) -> (95.825, 229.3849)
  line L65 (95.825, 229.3849) -> (95.825, 134.3849)
  line L66 (291, 321.3605) -> (291, 375) projected
  line L67 (291, 375) -> (79, 375) projected
  line L68 (79, 375) -> (79, 321.3605) projected
  point P0 (0, 0)
  dimension "d237" = 0
  dimension "d238" = 1
  dimension "d239" = 1
  dimension "d240" = 6
  dimension "d241" = 5
  constraints: 26 end point, 6 parallel, 4 horizontal, 3 perpendicular, 3 point on line, 1 point on circle
  measures "d237" distance between parallel lines of L32 L3
  measures "d238" distance between parallel lines of L31 L4
  measures "d239" distance between parallel lines of L30 L2
  measures "d240" distance of L57.start L57.end
  measures "d241" distance of L64.end L63.end
extrude "Выдавливание40" cut sketch "Эскиз46" against normal blind 10 contours A45 L64 L63 L62 A42 L22 | L22 A42 L65 A45 | L65 L23 L61 L25 | L61 A43 L24 A44 | A44 L24 A43 L58 L59 L60
fillet "Сопряжение4" radius 2 2 edges at (0.75, 375, -79) (0.75, 375, -291)
sketch "Эскиз47" plane through (1.5, 0, 0) normal (1, 0, 0) x (0, 0, -1)
  arc A0 (291, 373) -> (289, 375) centre (289, 373) ccw projected
  line L0 (289, 375) -> (81, 375) projected
  arc A1 (81, 375) -> (79, 373) centre (81, 373) ccw projected
  line L1 (79, 373) -> (79, 321.3605) projected
  arc A2 (78, 323.5966) -> (79, 321.3605) centre (81, 323.5966) ccw projected
  line L2 (78, 323.5966) -> (78, 372) projected
  arc A3 (78, 372) -> (75, 375) centre (75, 372) ccw projected
  line L3 (75, 375) -> (-15, 375) projected
  arc A4 (-15, 375) -> (-18, 372) centre (-15, 372) ccw projected
  line L4 (-18, 372) -> (-18, -2) projected
  arc A5 (-18, -2) -> (-15, -5) centre (-15, -2) ccw projected
  line L5 (-15, -5) -> (385, -5) projected
  arc A6 (385, -5) -> (388, -2) centre (385, -2) ccw projected
  line L6 (388, -2) -> (388, 372) projected
  arc A7 (388, 372) -> (385, 375) centre (385, 372) ccw projected
  line L7 (385, 375) -> (295, 375) projected
  arc A8 (295, 375) -> (292, 372) centre (295, 372) ccw projected
  line L8 (292, 372) -> (292, 323.5966) projected
  arc A9 (291, 321.3605) -> (292, 323.5966) centre (289, 323.5966) ccw projected
  line L9 (291, 321.3605) -> (291, 373) projected
  line L10 (100.825, 134.3849) -> (78.75, 134.3849) projected
  line L11 (78.75, 134.3849) -> (78.75, 229.3849) projected
  line L12 (78.75, 229.3849) -> (100.825, 229.3849) projected
  line L13 (100.825, 229.3849) -> (100.825, 134.3849) projected
  arc A10 (42, 27.152) -> (40, 25.152) centre (42, 25.152) ccw projected
  line L14 (40, 25.152) -> (40, 3) projected
  arc A11 (37, 0) -> (40, 3) centre (37, 3) ccw projected
  line L15 (37, 0) -> (-7, 0) projected
  arc A12 (-10, 3) -> (-7, 0) centre (-7, 3) ccw projected
  line L16 (-10, 3) -> (-10, 160) projected
  arc A13 (-7, 163) -> (-10, 160) centre (-7, 160) ccw projected
  line L17 (-7, 163) -> (37, 163) projected
  arc A14 (40, 160) -> (37, 163) centre (37, 160) ccw projected
  line L18 (40, 160) -> (40, 109.152) projected
  arc A15 (40, 109.152) -> (42, 107.152) centre (42, 109.152) ccw projected
  line L19 (42, 107.152) -> (54, 107.152) projected
  arc A16 (56, 105.152) -> (54, 107.152) centre (54, 105.152) ccw projected
  line L20 (56, 105.152) -> (56, 29.152) projected
  arc A17 (54, 27.152) -> (56, 29.152) centre (54, 29.152) ccw projected
  line L21 (54, 27.152) -> (42, 27.152) projected
  circle A18 centre (383.6, 368.9) radius 1.625 projected
  circle A19 centre (-13.6, 369) radius 1.625 projected
  circle A20 centre (383.6, 1.1) radius 1.625 projected
  circle A21 centre (-13.6, 1.1) radius 1.625 projected
  circle A22 centre (379.0468, 185.0848) radius 1.625 projected
  circle A23 centre (-9.0468, 185.0848) radius 1.625 projected
  circle A24 centre (379, 228) radius 1.625 projected
  circle A25 centre (-9, 228) radius 1.625 projected
  circle A26 centre (314.25, 368) radius 1.625 projected
  circle A27 centre (297.25, 228) radius 1.625 projected
  circle A28 centre (55.75, 228) radius 1.625 projected
  circle A29 centre (72.75, 142) radius 1.625 projected
  circle A30 centre (72.75, 2.0002) radius 1.625 projected
  circle A31 centre (55.75, 2.0002) radius 1.625 projected
  circle A32 centre (72.75, 368) radius 1.625 projected
  circle A33 centre (72.75, 228) radius 1.625 projected
  circle A34 centre (314.25, 142) radius 1.625 projected
  circle A35 centre (314.25, 228) radius 1.625 projected
  circle A36 centre (183.175, 129.0059) radius 1.85 projected
  circle A37 centre (297.25, 368) radius 1.625 projected
  circle A38 centre (314.25, 2.0002) radius 1.625 projected
  circle A39 centre (55.75, 142) radius 1.625 projected
  circle A40 centre (55.75, 368) radius 1.625 projected
  circle A41 centre (297.25, 2.0002) radius 1.625 projected
  circle A42 centre (297.25, 142) radius 1.625 projected
  arc A43 (185, 193.309) -> (185, 192.7028) centre (183.175, 193.0059) ccw projected
  line L22 (185, 193.309) -> (185, 192.7028) projected
  line L23 (14.5, 247.5001) -> (35, 247.5001) projected
  arc A44 (38, 244.5001) -> (35, 247.5001) centre (35, 244.5001) ccw projected
  line L24 (38, 244.5001) -> (38, 185.5001) projected
  arc A45 (35, 182.5001) -> (38, 185.5001) centre (35, 185.5001) ccw projected
  line L25 (35, 182.5001) -> (14.5, 182.5001) projected
  arc A46 (11.5, 185.5001) -> (14.5, 182.5001) centre (14.5, 185.5001) ccw projected
  line L26 (11.5, 185.5001) -> (11.5, 244.5001) projected
  arc A47 (14.5, 247.5001) -> (11.5, 244.5001) centre (14.5, 244.5001) ccw projected
  line L27 (358.5, 244.5001) -> (358.5, 185.5001) projected
  arc A48 (355.5, 182.5001) -> (358.5, 185.5001) centre (355.5, 185.5001) ccw projected
  line L28 (355.5, 182.5001) -> (335, 182.5001) projected
  arc A49 (332, 185.5001) -> (335, 182.5001) centre (335, 185.5001) ccw projected
  line L29 (332, 185.5001) -> (332, 244.5001) projected
  arc A50 (335, 247.5001) -> (332, 244.5001) centre (335, 244.5001) ccw projected
  line L30 (335, 247.5001) -> (355.5, 247.5001) projected
  arc A51 (358.5, 244.5001) -> (355.5, 247.5001) centre (355.5, 244.5001) ccw projected
  circle A52 centre (124.375, 129.0059) radius 2 projected
  circle A53 centre (124.375, 193.0059) radius 2 projected
  circle A54 centre (217.25, 312.9941) radius 2.1 projected
  circle A55 centre (152.75, 57.0059) radius 2.1 projected
  circle A56 centre (152.75, 118.0059) radius 2.1 projected
  circle A57 centre (152.75, 312.9941) radius 2.1 projected
  circle A58 centre (217.25, 251.9941) radius 2.1 projected
  circle A59 centre (217.25, 57.0059) radius 2.1 projected
  circle A60 centre (217.25, 118.0059) radius 2.1 projected
  circle A61 centre (152.75, 251.9941) radius 2.1 projected
  line L31 (165, 44) -> (165, 8) projected
  arc A62 (162, 5) -> (165, 8) centre (162, 8) ccw projected
  line L32 (162, 5) -> (96, 5) projected
  arc A63 (93, 8) -> (96, 5) centre (96, 8) ccw projected
  line L33 (93, 8) -> (93, 44) projected
  arc A64 (96, 47) -> (93, 44) centre (96, 44) ccw projected
  line L34 (96, 47) -> (162, 47) projected
  arc A65 (165, 44) -> (162, 47) centre (162, 44) ccw projected
  circle A66 centre (319.1128, 165.0002) radius 2.1 projected
  circle A67 centre (287, 56.343) radius 2.1 projected
  circle A68 centre (50.8872, 165.0002) radius 2.1 projected
  circle A69 centre (173.9908, 56.343) radius 2.1 projected
  circle A70 centre (135.25, 60) radius 2.1 projected
  circle A71 centre (103, 60) radius 2.1 projected
  arc A72 (40, 344.848) -> (42, 342.848) centre (42, 344.848) ccw projected
  line L35 (42, 342.848) -> (54, 342.848) projected
  arc A73 (56, 340.848) -> (54, 342.848) centre (54, 340.848) ccw projected
  line L36 (56, 340.848) -> (56, 264.848) projected
  arc A74 (54, 262.848) -> (56, 264.848) centre (54, 264.848) ccw projected
  line L37 (54, 262.848) -> (-8, 262.848) projected
  arc A75 (-10, 264.848) -> (-8, 262.848) centre (-8, 264.848) ccw projected
  line L38 (-10, 264.848) -> (-10, 367) projected
  arc A76 (-7, 370) -> (-10, 367) centre (-7, 367) ccw projected
  line L39 (-7, 370) -> (37, 370) projected
  arc A77 (40, 367) -> (37, 370) centre (37, 367) ccw projected
  line L40 (40, 367) -> (40, 344.848) projected
  line L41 (377, 0) -> (333, 0) projected
  arc A78 (330, 3) -> (333, 0) centre (333, 3) ccw projected
  line L42 (330, 3) -> (330, 28.152) projected
  arc A79 (330, 28.152) -> (327, 31.152) centre (327, 28.152) ccw projected
  line L43 (327, 31.152) -> (321, 31.152) projected
  arc A80 (318, 34.152) -> (321, 31.152) centre (321, 34.152) ccw projected
  line L44 (318, 34.152) -> (318, 100.152) projected
  arc A81 (321, 103.152) -> (318, 100.152) centre (321, 100.152) ccw projected
  line L45 (321, 103.152) -> (327, 103.152) projected
  arc A82 (327, 103.152) -> (330, 106.152) centre (327, 106.152) ccw projected
  line L46 (330, 106.152) -> (330, 160) projected
  arc A83 (333, 163) -> (330, 160) centre (333, 160) ccw projected
  line L47 (333, 163) -> (377, 163) projected
  arc A84 (380, 160) -> (377, 163) centre (377, 160) ccw projected
  line L48 (380, 160) -> (380, 3) projected
  arc A85 (377, 0) -> (380, 3) centre (377, 3) ccw projected
  line L49 (377, 266.848) -> (321, 266.848) projected
  arc A86 (318, 269.848) -> (321, 266.848) centre (321, 269.848) ccw projected
  line L50 (318, 269.848) -> (318, 335.848) projected
  arc A87 (321, 338.848) -> (318, 335.848) centre (321, 335.848) ccw projected
  line L51 (321, 338.848) -> (327, 338.848) projected
  arc A88 (327, 338.848) -> (330, 341.848) centre (327, 341.848) ccw projected
  line L52 (330, 341.848) -> (330, 367) projected
  arc A89 (333, 370) -> (330, 367) centre (333, 367) ccw projected
  line L53 (333, 370) -> (377, 370) projected
  arc A90 (380, 367) -> (377, 370) centre (377, 367) ccw projected
  line L54 (380, 367) -> (380, 269.848) projected
  arc A91 (377, 266.848) -> (380, 269.848) centre (377, 269.848) ccw projected
  line L55 (297.25, 2.0002) -> (297.25, 368)
  line L56 (297.25, 368) -> (72.75, 368)
  line L57 (72.75, 368) -> (72.75, 2.0002)
  line L58 (72.75, 2.0002) -> (297.25, 2.0002)
  line L59 (80.75, 10.0002) -> (80.75, 360)
  line L60 (80.75, 360) -> (289.25, 360)
  line L61 (289.25, 360) -> (289.25, 10.0002)
  line L62 (289.25, 10.0002) -> (80.75, 10.0002)
  line L63 (124.375, 129.0059) -> (183.175, 193.0059)
  line L64 (183.175, 193.0059) -> (217.25, 118.0059)
  line L65 (124.375, 193.0059) -> (217.25, 118.0059)
  line L66 (124.375, 129.0059) -> (124.375, 193.0059)
  line L67 (124.375, 193.0059) -> (183.175, 193.0059)
  line L68 (152.75, 251.9941) -> (183.175, 193.0059)
  line L69 (124.375, 193.0059) -> (152.75, 251.9941)
  line L70 (152.75, 251.9941) -> (217.25, 251.9941)
  line L71 (217.25, 251.9941) -> (152.75, 312.9941)
  line L72 (152.75, 312.9941) -> (217.25, 312.9941)
  line L73 (217.25, 312.9941) -> (217.25, 251.9941)
  line L74 (152.75, 251.9941) -> (152.75, 312.9941)
  line L75 (124.375, 193.0059) -> (152.75, 312.9941)
  line L76 (217.25, 118.0059) -> (217.25, 251.9941)
  line L77 (183.175, 193.0059) -> (217.25, 251.9941)
  line L78 (183.175, 129.0059) -> (217.25, 118.0059)
  line L79 (183.175, 129.0059) -> (183.175, 193.0059)
  line L80 (183.175, 129.0059) -> (124.375, 129.0059)
  line L81 (183.175, 129.0059) -> (152.75, 118.0059)
  line L82 (124.375, 129.0059) -> (152.75, 118.0059)
  line L83 (152.75, 118.0059) -> (217.25, 118.0059)
  line L84 (135.25, 60) -> (103, 60)
  line L85 (124.375, 129.0059) -> (103, 60)
  line L86 (217.25, 57.0059) -> (124.375, 129.0059)
  line L87 (124.375, 129.0059) -> (152.75, 57.0059)
  line L88 (217.25, 57.0059) -> (217.25, 118.0059)
  line L89 (135.25, 60) -> (152.75, 57.0059)
  line L90 (173.9908, 56.343) -> (152.75, 57.0059)
  line L91 (152.75, 57.0059) -> (152.75, 118.0059)
  line L92 (173.9908, 56.343) -> (217.25, 57.0059)
  line L93 (173.9908, 56.343) -> (152.75, 118.0059)
  line L94 (135.25, 60) -> (124.375, 129.0059)
  point P0 (0, 0)
  dimension "d252" = 8
  constraints: 80 end point, 8 perpendicular, 6 parallel, 4 vertical, 1 horizontal, 3 other
  measures "d252" distance between parallel lines of L57 L59